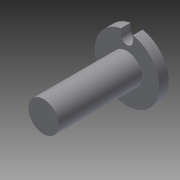
# Autodesk Inventor part: pulley shaft
Saved by Autodesk Inventor 2015 (Build 190159000, 159)
## iProperties
Created: 2016-02-13
Part Number: pulley shaft
Material: Generic
Document SubType Name: Modeling
Designer: Owner
Density: 1 g/cm^3
Appearance: Default
Mass: 1.66006 g
Surface Area: 11.3717 cm^2
Volume: 1.66006 cm^3
Author: Owner
Autodesk Inventor part; units mm, degrees
ref_plane "YZ Plane" through (0, 0, 0) normal (1, 0, 0) x (0, 1, 0)
ref_plane "XZ Plane" through (0, 0, 0) normal (0, 1, 0) x (-1, 0, 0)
ref_plane "XY Plane" through (0, 0, 0) normal (0, 0, 1) x (1, 0, 0)
sketch "Sketch1" plane through (0, 0, 0) normal (0, 0, 1) x (1, 0, 0)
  circle A0 centre (0, 0) radius 8.509
  dimension "d0" = 17.018
  constraints: 1 centre point, 1 coincident
  measures "d0" diameter of A0
extrude "Extrusion1" add sketch "Sketch1" along normal blind 2.54
sketch "Sketch3" plane through (0, 0, 0) normal (0, 0, -1) x (-1, 0, 0)
  line L0 (0, 0) -> (0, 6.9342)
  circle A0 centre (0, 6.9342) radius 1.5875
  line L1 (-1.5875, 6.9342) -> (-1.5875, 8.3596)
  circle A1 centre (0, 0) radius 8.509 projected
  line L2 (1.5875, 6.9342) -> (1.5875, 8.3596)
  dimension "d6" = 6.9342
  dimension "d7" = 3.175
  constraints: 6 end point, 4 point on circle, 2 tangent, 2 vertical, 1 centre point, 1 coincident, 1 parallel
  measures "d6" distance of L0.start L0.end
  measures "d7" diameter of A0
extrude "Extrusion3" cut sketch "Sketch3" against normal through all contours A0 A1 | A0 A1 L2 | A0 L1 A1 picked at (-0.1424, 6.414)
sketch "Sketch2" plane through (0, 0, 2.54) normal (0, 0, 1) x (1, 0, 0)
  circle A0 centre (0, 0) radius 8.509 projected
  circle A1 centre (0, 0) radius 4.0005
  dimension "d3" = 8.001
  constraints: 1 centre point, 1 coincident
  measures "d3" diameter of A1
extrude "Extrusion2" add sketch "Sketch2" along normal blind 21.971 contours A1
body "Solid1"
